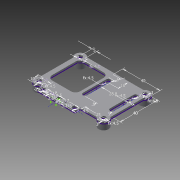
# Autodesk Inventor part: Bar
Saved by Autodesk Inventor 2014 SP1 (Build 180222100, 222)
## iProperties
Created: 2015-03-26
Part Number: Bar
Material: Generic
Document SubType Name: Modeling
Designer: Erin
Density: 1 g/cm^3
Appearance: Default
Author: Erin
Autodesk Inventor part; units mm, degrees
ref_plane "YZ Plane" through (0, 0, 0) normal (1, 0, 0) x (0, 1, 0)
ref_plane "XZ Plane" through (0, 0, 0) normal (0, 1, 0) x (-1, 0, 0)
ref_plane "XY Plane" through (0, 0, 0) normal (0, 0, 1) x (1, 0, 0)
sketch "Sketch1" plane through (0, 0, 0) normal (0, 0, 1) x (1, 0, 0)
  line L0 (-20, -3) -> (20, -3) construction
  circle A0 centre (-17, 0) radius 2.25
  circle A1 centre (17, 0) radius 2.25
  circle A2 centre (0, 0) radius 2.25
  circle A3 centre (-7, 0.3446) radius 1
  circle A4 centre (7, 0.3446) radius 1
  line L1 (-23.9554, 0) -> (25.6733, 0) construction
  line L2 (0, 11.421) -> (0, -11.2937) construction
  line L3 (-20, -3) -> (20, -3)
  line L4 (20, -3) -> (20, 3)
  line L5 (20, 3) -> (-20, 3)
  line L6 (-20, 3) -> (-20, -3)
  circle A5 centre (-11.8345, 1.6861) radius 0.5
  line L7 (-30, 3) -> (45, 3)
  line L8 (45, 3) -> (45, 13)
  line L9 (45, 13) -> (-30, 13)
  line L10 (-30, 13) -> (-30, 3)
  line L11 (-30, 13) -> (-25, 13)
  line L12 (-25, 13) -> (-25, 48)
  line L13 (-25, 53) -> (-30, 53)
  line L14 (-30, 53) -> (-30, 13)
  line L15 (45, 13) -> (5, 13)
  line L16 (5, 13) -> (5, 48)
  line L17 (5, 53) -> (45, 53)
  line L18 (45, 53) -> (45, 13)
  line L19 (10.1, 13) -> (10.1, 53) construction
  line L20 (39, 13) -> (39, 53) construction
  line L21 (10.1, 18) -> (10.1, 43) construction
  line L22 (12.35, 18) -> (12.35, 43)
  line L23 (7.85, 43) -> (7.85, 18)
  arc A6 (7.85, 18) -> (12.35, 18) centre (10.1, 18) ccw
  arc A7 (12.35, 43) -> (7.85, 43) centre (10.1, 43) ccw
  line L24 (39, 18) -> (39, 43) construction
  line L25 (41.25, 18) -> (41.25, 43)
  line L26 (36.75, 43) -> (36.75, 18)
  arc A8 (36.75, 18) -> (41.25, 18) centre (39, 18) ccw
  arc A9 (41.25, 43) -> (36.75, 43) centre (39, 43) ccw
  line L27 (-25, 53) -> (5, 53)
  line L28 (5, 53) -> (5, 48)
  line L29 (5, 48) -> (-25, 48)
  line L30 (-25, 48) -> (-25, 53)
  line L31 (-25, 48) -> (-25, 53)
  line L32 (5, 48) -> (5, 53)
  circle A10 centre (-27, 50) radius 2.25
  circle A11 centre (-27, 6) radius 2.25
  circle A12 centre (42, 50) radius 2.25
  circle A13 centre (42, 6) radius 2.25
  circle A14 centre (-27, 50) radius 5.25
  circle A15 centre (42, 50) radius 5.25
  circle A16 centre (42, 6) radius 5.25
  circle A17 centre (-27, 6) radius 5.25
  point P0 (0, 0)
  point P1 (0, -3)
  point P2 (0, -3)
  point P3 (-2.8751, -5.808)
  point P4 (2.8751, -5.808)
  point P5 (10.1, 30.5)
  point P6 (39, 30.5)
  dimension "d0" = 40
  dimension "d1" = 4.5
  dimension "d2" = 4.5
  dimension "d3" = 3
  dimension "d4" = 4.5
  dimension "d5" = 3
  dimension "d6" = 3.3446
  dimension "d7" = 3.3446
  dimension "d8" = 3
  dimension "d9" = 17
  dimension "d10" = 17
  dimension "d11" = 3
  dimension "d12" = 3
  dimension "d13" = 3
  dimension "d14" = 3
  dimension "d16" = 1
  dimension "d20" = 10
  dimension "d21" = 25
  dimension "d22" = 10
  dimension "d23" = 5
  dimension "d25" = 40
  dimension "d26" = 40
  dimension "d30" = 4.5
  dimension "d31" = 5
  dimension "d32" = 10
  dimension "d33" = 4.5
  dimension "d34" = 5
  dimension "d35" = 10
  dimension "d36" = 5
  dimension "d37" = 28.9
  dimension "d38" = 6
  dimension "d40" = 4.5
  dimension "d41" = 3
  dimension "d42" = 3
  dimension "d43" = 4.5
  dimension "d44" = 3
  dimension "d45" = 3
  dimension "d46" = 4.5
  dimension "d47" = 3
  dimension "d48" = 3
  dimension "d49" = 4.5
  dimension "d50" = 3
  dimension "d51" = 3
  dimension "d54" = 3
  dimension "d55" = 3
  dimension "d57" = 3
  dimension "d58" = 3
  constraints: 70 end point, 18 centre point, 15 parallel, 10 perpendicular, 10 point on line, 8 point on circle, 8 tangent, 6 horizontal, 5 coincident, 3 midpoint, 2 collinear, 1 vertical
  measures "d0" distance of L0.start L0.end
  measures "d1" diameter of A0
  measures "d2" diameter of A1
  measures "d3" distance from line of A0.centre L0
  measures "d4" diameter of A2
  measures "d5" distance from line of A2.centre L0
  measures "d6" distance from line of A3.centre L0
  measures "d7" distance from line of A4.centre L0
  measures "d8" distance between parallel lines of L0 L1
  measures "d9" distance from line of L2 A1.centre
  measures "d10" distance from line of L2 A0.centre
  measures "d11" distance from line of A0.centre L3
  measures "d12" distance from line of A0.centre L6
  measures "d13" distance from line of A0.centre L5
  measures "d14" distance from line of A1.centre L4
  measures "d16" diameter of A5
  measures "d20" distance of L9.end L7.start
  measures "d21" distance between parallel lines of L4 L8
  measures "d22" distance between parallel lines of L6 L10
  measures "d23" distance of L13.end L13.start
  measures "d25" distance of L17.end L8.end
  measures "d26" distance of L17.start L17.end
  measures "d30" diameter of A7
  measures "d31" distance from line of L9 L21.start
  measures "d32" distance from line of L21.end L17
  measures "d33" diameter of A9
  measures "d34" distance from line of L24.start L9
  measures "d35" distance from line of L24.end L17
  measures "d36" distance of L27.end L16.end
  measures "d37" distance between parallel lines of L21 L20
  measures "d38" distance between parallel lines of L18 L24
  measures "d40" diameter of A10
  measures "d41" distance from line of A10.centre L13
  measures "d42" distance from line of A10.centre L14
  measures "d43" diameter of A11
  measures "d44" distance from line of A11.centre L7
  measures "d45" distance from line of A11.centre L10
  measures "d46" diameter of A12
  measures "d47" distance from line of A12.centre L18
  measures "d48" distance from line of A12.centre L17
  measures "d49" diameter of A13
  measures "d50" distance from line of A13.centre L7
  measures "d51" distance from line of A13.centre L8
  measures "d54" radial gap between concentric circles of A10 A14
  measures "d55" radial gap between concentric circles of A12 A15
  measures "d57" radial gap between concentric circles of A13 A16
  measures "d58" radial gap between concentric circles of A11 A17
extrude "Extrusion1" add sketch "Sketch1" along normal blind 2 contours L6 L5 L4 L3 | L7 A17 L10 L9 L8 A16 L5 | L7 L10 A17 | A16 L8 L7 | L14 A14 L12 L9 | L9 L16 L28 L17 A15 L18 | L14 L13 L30 A10 L12 A14 | A15 L17 L18 | A14 L29 L30 A10 L27 | L27 L28 L29 A14 | A10 L30 | L30 A10 | A11 | A12 | A13 picked at (-26.4735, 3.2555) picked at (41.4735, 3.2555) picked at (41.4735, 52.7445)
fillet "Fillet1" radius 1 2 edges at (-20, -3, 1) (20, -3, 1)
fillet "Fillet2" radius 5 8 edges at (-30, 3, 1) (45, 3, 1) (45, 53, 1) (-30, 53, 1) (-25, 48, 1) (-25, 13, 1) (5, 13, 1) (5, 48, 1)
extrude "Extrusion2" cut sketch "Sketch1" along normal blind 10 contours A10 L30 | L30 A10 | A11 | A12 | A13
extrude "Extrusion3" add sketch "Sketch1" along normal blind 2 contours A17 L10 L7 | L7 L10 A17 | A16 L8 L7 | L7 L8 A16 | A14 L27 L13 L14 | L14 L13 L30 A10 L12 A14 | A15 L17 L18 | L18 L17 A15 | L12 L29 A14 | A14 L29 L30 A10 L27
extrude "Extrusion4" add sketch "Sketch1" against normal blind 6 contours A17 L10 L7 | L7 L10 A17 | A16 L8 L7 | L7 L8 A16 | A14 L27 L13 L14 | L14 L13 L30 A10 L12 A14 | A15 L17 L18 | L18 L17 A15 | L12 L29 A14 | A14 L29 L30 A10 L27
equation "\"d30\" = screw"
equation "\"d33\" = screw"
equation "\"d40\" = screw"
equation "\"d43\" = screw"
equation "\"d46\" = screw"
equation "\"d49\" = screw"
equation "\"screw\" = 4.5"
body "Solid1"
